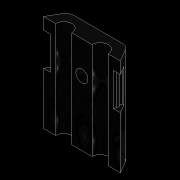
# Autodesk Inventor part: 3d_LM - Pinza 1
Saved by Autodesk Inventor 2018.3 (Build 223284000, 284)
## iProperties
Created: 2026-02-09
Part Number: 3d_LM - Pinza 1
Material: PA12 SLS 3D Print
Document SubType Name: Modeling
Designer: aca6
Density: 0.95 g/cm^3
Appearance: Black
Author: aca6
Comments: DIN-ISO-2768-mK
Autodesk Inventor part; units mm, degrees
ref_plane "YZ Plane" through (0, 0, 0) normal (1, 0, 0) x (0, 1, 0)
ref_plane "XZ Plane" through (0, 0, 0) normal (0, 1, 0) x (-1, 0, 0)
ref_plane "XY Plane" through (0, 0, 0) normal (0, 0, 1) x (1, 0, 0)
sketch "Sketch1" plane through (0, 0, 0) normal (0, 0, 1) x (1, 0, 0)
  line L0 (-4.752, -2.1513) -> (-3.25, -2.1513)
  arc A0 (-1.25, -2.1513) -> (-3.25, -2.1513) centre (-2.25, -2.1513) ccw
  line L1 (-3.25, -2.1513) -> (1.2966, -2.1513) construction
  line L2 (-1.25, -2.1513) -> (1.25, -2.1513)
  arc A1 (3.25, -2.1513) -> (1.25, -2.1513) centre (2.25, -2.1513) ccw
  line L3 (1.25, -2.1513) -> (6.8796, -2.1513) construction
  line L4 (3.25, -2.1513) -> (4.752, -2.1513)
  line L5 (-4.752, -2.1513) -> (-3.886, -0.6513)
  line L6 (-4.752, -2.1513) -> (-3.02, -2.1513) construction
  arc A2 (-3.02, -0.1513) -> (-3.886, -0.6513) centre (-3.02, -1.1513) ccw
  line L7 (-3.886, -0.6513) -> (-3.02, -0.1513) construction
  line L8 (-3.02, -0.1513) -> (3.02, -0.1513)
  line L9 (4.752, -2.1513) -> (3.886, -0.6513)
  line L10 (4.752, -2.1513) -> (6.484, -2.1513) construction
  arc A3 (3.886, -0.6513) -> (3.02, -0.1513) centre (3.02, -1.1513) ccw
  line L11 (0, 0) -> (0, 1.588) construction
  dimension "d1" = 2
  dimension "d2" = 2.5
  dimension "d3" = 2
  dimension "d5" = 60
  dimension "d6" = 1.732
  dimension "d7" = 1
  dimension "d8" = 1
  dimension "d9" = 6.04
  dimension "d10" = 1.732
  dimension "d11" = 120
  dimension "d12" = 1
  dimension "d34" = 9.504
  dimension "d35" = 1.502
  dimension "d36" = 1.502
  constraints: 24 end point, 8 horizontal, 8 point on circle, 4 centre point, 4 point on line, 2 equal length, 2 tangent, 2 vertical, 1 horizontal alignment, 1 symmetric about line, 2 other
  measures "d1" diameter of A0
  measures "d2" distance of L2.start L2.end
  measures "d3" diameter of A1
  measures "d5" angle of L6 L5
  measures "d6" distance of L0.start L5.end
  measures "d7" radius of A2
  measures "d8" distance of L5.end L7.end
  measures "d9" distance of L7.end L8.end
  measures "d10" distance of L4.end L9.end
  measures "d11" angle of L10 L9
  measures "d12" radius of A3
  measures "d34" distance of L4.end L0.start
  measures "d35" distance of L0.start L0.end
  measures "d36" distance of L4.end L4.start
extrude "Extrusion1" add sketch "Sketch1" along normal blind 12
sketch "Sketch2" plane through (-3.02, -0.1513, 0) normal (0, 1, 0) x (1, 0, 0)
  line L0 (6.04, -12) -> (0, -12) projected
  line L1 (7.772, 0) -> (7.772, -12) projected
  point P0 (3.02, 0)
  point P1 (3.02, -8)
  dimension "d22" = 4
  dimension "d23" = 4.752
  measures "d22" distance from line of L0 point (3.02, -8)
  measures "d23" distance from line of L1 point (3.02, -8)
hole "Hole1" at (0, -0.1513, 8) direction (0, -1, 0) diameter 1.5 depth 8 tip angle 118
ref_plane "Work Plane1" through (0, 0, 10.55) normal (0, 0, 1) x (1, 0, 0)
sketch "Sketch3" plane through (0, 0, 10.55) normal (0, 0, 1) x (1, 0, 0)
  line L0 (-4.1458, -1.1013) -> (-3.9448, -1.1013)
  line L1 (-4.752, -2.1513) -> (-3.25, -2.1513) projected
  line L2 (-3.886, -0.6513) -> (-4.752, -2.1513) projected
  line L3 (-3.9448, -1.1013) -> (-3.6515, -1.5013)
  line L4 (-3.6515, -1.5013) -> (-4.0005, -1.5013)
  line L5 (-4.0005, -1.5013) -> (-4.0005, -1.8513)
  line L6 (-4.0005, -1.8513) -> (-3.8913, -2.1513)
  line L7 (-4.1458, -1.1013) -> (-4.752, -2.1513)
  line L8 (-4.752, -2.1513) -> (-3.8913, -2.1513)
  point P0 (0, 0)
  dimension "d25" = 1.05
  dimension "d26" = 0.201
  dimension "d27" = 126.25
  dimension "d28" = 0.496
  dimension "d29" = 0.349
  dimension "d30" = 0.35
  dimension "d31" = 160
  constraints: 14 end point, 2 collinear, 2 horizontal, 2 point on line, 1 vertical
  measures "d25" distance between parallel lines of L1 L0
  measures "d26" distance of L0.start L0.end
  measures "d27" angle of L0 L3
  measures "d28" distance of L0.end L3.end
  measures "d29" distance of L3.end L4.end
  measures "d30" distance of L4.end L5.end
  measures "d31" angle of L5 L6
extrude "Extrusion2" cut sketch "Sketch3" against normal blind 4.1
mirror "Mirror1" about plane through (0, 0, 0) normal (1, 0, 0) of "Extrusion2"
body "Solid1"
